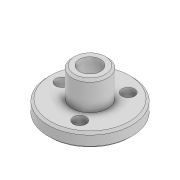
# Autodesk Inventor part: Nut
Saved by Autodesk Inventor 2020 (Build 240168000, 168)
## iProperties
Created: 2022-06-16
Part Number: Nut
Material: Generic
Document SubType Name: Modeling
Designer: ferrerx
Density: 1 g/cm^3
Appearance: Default
Author: ferrerx
Autodesk Inventor part; units mm, degrees
ref_plane "YZ Plane" through (0, 0, 0) normal (1, 0, 0) x (0, 1, 0)
ref_plane "XZ Plane" through (0, 0, 0) normal (0, 1, 0) x (-1, 0, 0)
ref_plane "XY Plane" through (0, 0, 0) normal (0, 0, 1) x (1, 0, 0)
sketch "Sketch1" plane through (0, 0, 0) normal (0, 1, 0) x (-1, 0, 0)
  circle A0 centre (0, 0) radius 9.5
  circle A1 centre (0, 0) radius 2.4
  dimension "d0" = 19
  dimension "d1" = 4.8
  constraints: 2 centre point, 2 coincident
  measures "d0" diameter of A0
  measures "d1" diameter of A1
extrude "Extrusion1" add sketch "Sketch1" along normal blind 3.18
sketch "Sketch2" plane through (0, 3.18, 0) normal (0, 1, 0) x (1, 0, 0)
  circle A0 centre (0, 0) radius 2.4
  circle A1 centre (0, 0) radius 4
  circle A2 centre (0, 0) radius 2.4 projected
  dimension "d4" = 8
  constraints: 2 centre point, 2 coincident, 1 concentric
  measures "d4" diameter of A1
extrude "Extrusion2" add sketch "Sketch2" along normal blind 6.5
sketch "Sketch3" plane through (0, 3.18, 0) normal (0, 1, 0) x (1, 0, 0)
  circle A0 centre (-6.35, 0) radius 1.45
  circle A1 centre (0, 0) radius 6.35 construction
  dimension "d8" = 12.7
  dimension "d7" = 2.9
  constraints: 1 centre point, 1 coincident, 1 horizontal alignment, 2 other
  measures "d7" diameter of A0
extrude "Extrusion3" cut sketch "Sketch3" against normal blind 6.5
pattern_circular "Circular Pattern1" count 3 over 360 about axis through (0, 3.18, 0) along (0, 1, 0) of "Extrusion3"
chamfer "Chamfer1" distance 0.5 angle 45 3 edges at (-4, 9.68, 0) (9.5, 3.18, 0) (9.5, 0, 0)
body "Solid1"
